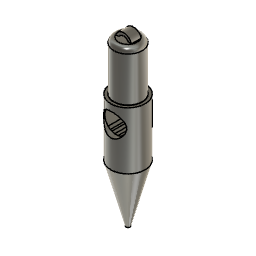
test nose cone v4 (Autodesk Fusion 360 design; units mm, degrees)
Autodesk Fusion 360 part; units mm, degrees
note: some values were not read from the file. Chosen so that the rebuilt part matches the saved one: which bodies a step acts on. Set by a fixed rule: which sketch regions a step uses.
sketch "Sketch1" plane through (0, 0, 0) normal (0, 1, 0) x (1, 0, 0)
  line L0 (-30, 466.4818) -> (-17.5, 473.5668)
  line L1 (0, 380) -> (0, 382.9635)
  line L2 (-14.4962, 382.9635) -> (0, 382.9635)
  line L3 (0, 550) -> (0, 382.9635)
  line L4 (-12.0481, 512.1856) -> (-35.0172, 529.9796)
  line L5 (-14.4962, 433) -> (-14.4962, 382.9635)
  line L6 (-18.356, 433) -> (-18.3, 433)
  line L7 (-17.5, 433.3365) -> (-14.5, 433.3365)
  arc A0 (-18.3, 433) -> (-18.5, 432.8) centre (-18.3, 432.8) ccw
  line L8 (-14.4962, 382.9635) -> (-14.4962, 433)
  line L9 (0, 382.9635) -> (0, 380)
  line L10 (17.5, 233) -> (-17.5, 233)
  line L11 (-14.4962, 397.7519) -> (-14.4962, 382.9635)
  line L12 (0, 382.9635) -> (0, 405)
  line L13 (-17.5, 433.3365) -> (-14.5, 433.3365)
  line L14 (-14.5, 433.3365) -> (-14.4962, 433)
  line L15 (0, 550) -> (-2, 550)
  line L16 (0, 550) -> (-2, 550)
  line L17 (-17.5, 456.7981) -> (-30, 466.4818)
  line L18 (0, 483.4858) -> (14.4363, 491.6682)
  line L19 (0, 382.9635) -> (-14.4962, 382.9635)
  line L20 (14.4363, 491.6682) -> (0, 502.8519)
  line L21 (-17.5, 433.3365) -> (-17.5, 491.6682)
  line L22 (-17.5, 491.6682) -> (-2, 550)
  line L23 (-14.4962, 382.9635) -> (-90, 460)
  line L24 (-90, 460) -> (-45.5915, 565.8682)
  line L25 (-45.5915, 565.8682) -> (-2, 550)
  constraint perpendicular L7 L21
  constraint coincident L21 L17.start
  constraint coincident L21 L0.end
  constraint coincident L22 L4.start
revolve "Revolve1" add sketch "Sketch1" angle 360 about axis through (0, 0, -382.9635) along (0, 0, 1) contours L2 L3 L5 L7 L8 L11 L12 L13 L14 L15 L16 L19 L21 L22 makes body 1
fillet "Fillet1" [no effect]
fillet "Fillet2" radius 5 1 edges at (-13.5152, 5.242, -382.9635) on bodies 1
ref_plane "WorkPlane1" through (0, 0, -382.9635) normal (0, 0, 1) x (1, 0, 0)
ref_plane "WorkPlane2" through (0, -14.4962, -421.9536) normal (0, -1, 0) x (1, 0, 0)
ref_plane "WorkPlane3" through (0, 0.5038, -421.9536) normal (0, -1, 0) x (1, 0, 0)
sketch "Sketch2" plane through (0, 0.5038, -421.9536) normal (0, -1, 0) x (1, 0, 0)
  arc A0 (5, 39) -> (-5, 39) centre (0, 36.3333) ccw
  arc A1 (8, 39) -> (-8, 39) centre (0, 36.6667) ccw
  line L0 (-8, 39) -> (-5, 39)
  line L1 (5, 39) -> (8, 39)
  constraint horizontal L0
  constraint parallel L0 L1
extrude "Extrude1" add sketch "Sketch2" along normal mid plane 10 separate body makes body 2
combine "Combine1" operation add target body 2 tool bodies 1 makes body 3 at (-17.4782, 0.8723, -452.7804)
combine "Combine2" operation add target body 2 tool bodies 3 makes body 4 at (-17.4782, 0.8723, -452.7804)
extrude "Extrude2" add 2 faces at (7, -1.1628, -382.9536) (-6, -1.1628, -382.9536) along direction (0, 0, -1) blind 5 on bodies 2 bodies 2 4
sketch "Sketch3" plane through (0, -14.4962, -421.9536) normal (0, -1, 0) x (1, 0, 0)
  line L0 (1.65, -43.7503) -> (7.65, -43.7503)
  line L1 (7.65, -41.5) -> (11.75, -41.5)
  line L2 (7.65, -43.7503) -> (7.65, -41.5)
  line L3 (1.65, -41.5) -> (1.65, -43.7503)
  line L4 (11.75, -41.5) -> (11.75, -18)
  line L5 (11.75, -18) -> (-11.75, -18)
  line L6 (-11.75, -18) -> (-11.75, -41.5)
  line L7 (-7.65, -41.5) -> (-7.65, -43.7503)
  line L8 (-15.75, -14) -> (15.75, -14)
  line L9 (-7.65, -43.7503) -> (-1.65, -43.7503)
  line L10 (15.75, -14) -> (15.75, -45.5)
  line L11 (-11.75, -41.5) -> (-7.65, -41.5)
  line L12 (-1.65, -43.7503) -> (-1.65, -41.5)
  line L13 (-15.75, -45.5) -> (-15.75, -14)
  line L14 (-1.65, -41.5) -> (1.65, -41.5)
  line L15 (15.75, -45.5) -> (-15.75, -45.5)
extrude "Extrude3" cut sketch "Sketch3" against normal blind 50 contours L0 L1 L2 L3 L4 L5 L6 L7 L9 L11 L12 L14 bodies 2
extrude "Extrude4" cut sketch "Sketch3" along normal blind 10 contours L0 L1 L2 L3 L4 L5 L6 L7 L9 L11 L12 L14 bodies 2
ref_plane "WorkPlane4" through (11.75, -12.9687, -439.9536) normal (0, -1, 0) x (1, 0, 0)
sketch "Sketch4" plane through (11.75, -12.9687, -439.9536) normal (0, -1, 0) x (1, 0, 0)
  line L0 (-23.5, -23.5) -> (-19.4, -23.5)
  line L1 (-23.5, -23.5) -> (-23.5, 0)
  line L2 (0, 0) -> (-23.5, 0)
  line L3 (0, 0) -> (0, -23.5)
  line L4 (-4.1, -23.5) -> (0, -23.5)
  line L5 (-4.1, -23.5) -> (-4.1, -25.7503)
  line L6 (-10.1, -25.7503) -> (-4.1, -25.7503)
  line L7 (-10.1, -25.7503) -> (-10.1, -23.5)
  line L8 (-13.4, -23.5) -> (-10.1, -23.5)
  line L9 (-13.4, -23.5) -> (-13.4, -25.7503)
  line L10 (-19.4, -25.7503) -> (-13.4, -25.7503)
  line L11 (-19.4, -25.7503) -> (-19.4, -23.5)
  line L12 (-10.1, -23.5) -> (-10.1, -25.7503)
  line L13 (-10.1, -25.7503) -> (-4.1, -25.7503)
  line L14 (-4.1, -25.7503) -> (-4.1, -23.5)
  line L15 (-4.1, -23.5) -> (0, -23.5)
  line L16 (0, -23.5) -> (0, 0)
  line L17 (0, 0) -> (-23.5, 0)
  line L18 (-23.5, 0) -> (-23.5, -23.5)
  line L19 (-23.5, -23.5) -> (-19.4, -23.5)
  line L20 (-19.4, -23.5) -> (-19.4, -25.7503)
  line L21 (-19.4, -25.7503) -> (-13.4, -25.7503)
  line L22 (-13.4, -25.7503) -> (-13.4, -23.5)
  line L23 (-13.4, -23.5) -> (-10.1, -23.5)
  line L24 (-29.25, 6.6171) -> (5.75, 6.6171)
  line L25 (-29.25, -51.7146) -> (5.75, -51.7146)
  line L26 (-23.5, 0) -> (0, 0)
  line L27 (0, 0) -> (0, -23.5)
  line L28 (0, -23.5) -> (-23.5, -23.5)
  line L29 (-23.5, -23.5) -> (-23.5, 0)
  line L30 (-23.5, 0) -> (-11.75, 0)
  line L31 (-11.75, 0) -> (-11.75, -23.5)
  circle A0 centre (-11.75, -11.75) radius 11.75
  constraint horizontal L26
  constraint vertical L27
  constraint horizontal L28
  constraint vertical L29
  constraint coincident L3.end L4.end
  constraint coincident L1.end L2.end
  constraint midpoint L26 L30.end
  constraint midpoint L8 L31.end
  constraint midpoint L31 A0.centre
  constraint coincident L30.end A0
extrude "Extrude5" add sketch "Sketch4" along normal blind 5 contours L0 L1 L8 L18 L19 L23 L28 L29 A0 | L9 L10 L11 L20 L21 L22 L28 | L1 L2 L17 L18 L26 L29 L30 A0 | L2 L3 L16 L17 L26 L27 A0 | L3 L4 L8 L15 L16 L23 L27 L28 A0 | L5 L6 L7 L12 L13 L14 L28 bodies 2
revolve "Revolve2" cut sketch "Sketch1" angle 360 about axis through (0, 0, -550) along (0, 0, 1) contours L0 L5 L7 L8 L11 L13 L14 L17 L21 L22 L23 L24 L25 | L0 L17 L21 bodies 2
extrude "Extrude6" add 4 faces at (10.8955, -12.9687, -459.7604) (-10.8955, -12.9687, -459.7604) (-9.4208, -12.9687, -442.2827) (9.4208, -12.9687, -442.2827) along direction (0, 1, 0) blind 1 on bodies 2 bodies 2
ref_plane "WorkPlane5" through (-5.875, 11.0313, -445.8286) normal (0, 1, 0) x (-1, 0, 0)
sketch "Sketch5" plane through (-5.875, 11.0313, -445.8286) normal (0, 1, 0) x (1, 0, 0)
  spline S0 degree 3 poles (5.875, -5.875) (5.1105, -5.875) (4.3276, -5.7992) (2.786, -5.4889) (2.0272, -5.2546) (-0.1352, -4.342) (-1.4233, -3.4437) (-3.4554, -1.4116) (-4.346, -0.1261) (-5.2531, 2.0237) (-5.4866, 2.7777) (-5.7976, 4.3166) (-5.875, 5.1016) (-5.875, 5.875) knots -1.845512 -1.845512 -1.845512 -1.845512 -1.616148 -1.616148 -1.386784 -1.386784 -0.928056 -0.928056 -0.464028 -0.464028 -0.232014 -0.232014 0 0 0 0
  spline S1 degree 3 poles (17.625, 5.875) (17.625, 5.1016) (17.5476, 4.3166) (17.2366, 2.7777) (17.0031, 2.0237) (16.096, -0.1261) (15.2054, -1.4116) (13.1733, -3.4437) (11.8852, -4.342) (9.7228, -5.2546) (8.964, -5.4889) (7.4224, -5.7992) (6.6395, -5.875) (5.875, -5.875) knots -3.691025 -3.691025 -3.691025 -3.691025 -3.459011 -3.459011 -3.226997 -3.226997 -2.762969 -2.762969 -2.304241 -2.304241 -2.074877 -2.074877 -1.845512 -1.845512 -1.845512 -1.845512
  spline S2 degree 3 poles (5.875, 17.625) (6.6395, 17.625) (7.4224, 17.5492) (8.964, 17.2389) (9.7228, 17.0046) (11.8852, 16.092) (13.1733, 15.1937) (15.2054, 13.1616) (16.096, 11.8761) (17.0031, 9.7263) (17.2366, 8.9723) (17.5476, 7.4334) (17.625, 6.6484) (17.625, 5.875) knots 1.845512 1.845512 1.845512 1.845512 2.074877 2.074877 2.304241 2.304241 2.762969 2.762969 3.226997 3.226997 3.459011 3.459011 3.691025 3.691025 3.691025 3.691025
  spline S3 degree 3 poles (-5.875, 5.875) (-5.875, 6.6484) (-5.7976, 7.4334) (-5.4866, 8.9723) (-5.2531, 9.7263) (-4.346, 11.8761) (-3.4554, 13.1616) (-1.4233, 15.1937) (-0.1352, 16.092) (2.0272, 17.0046) (2.786, 17.2389) (4.3276, 17.5492) (5.1105, 17.625) (5.875, 17.625) knots 0 0 0 0 0.232014 0.232014 0.464028 0.464028 0.928056 0.928056 1.386784 1.386784 1.616148 1.616148 1.845512 1.845512 1.845512 1.845512
  line L0 (7.525, 17.625) -> (7.525, 19.8753)
  line L1 (13.525, 19.8753) -> (7.525, 19.8753)
  line L2 (13.525, 19.8753) -> (13.525, 17.625)
  line L3 (17.625, 17.625) -> (13.525, 17.625)
  line L4 (17.625, 17.625) -> (17.625, -5.875)
  line L5 (-5.875, -5.875) -> (17.625, -5.875)
  line L6 (-5.875, -5.875) -> (-5.875, 17.625)
  line L7 (-1.775, 17.625) -> (-5.875, 17.625)
  line L8 (-1.775, 17.625) -> (-1.775, 19.8753)
  line L9 (4.225, 19.8753) -> (-1.775, 19.8753)
  line L10 (4.225, 19.8753) -> (4.225, 17.625)
  line L11 (7.525, 17.625) -> (4.225, 17.625)
  line L12 (23.375, -12.4921) -> (-11.625, -12.4921)
  line L13 (23.375, 45.8396) -> (-11.625, 45.8396)
extrude "Extrude7" add sketch "Sketch5" along normal blind 10 separate body makes body 5
sketch "Sketch6" plane through (0, 0, -433.3365) normal (0, 0, 1) x (-1, 0, 0)
  circle A0 centre (0, 0) radius 14.5
  circle A1 centre (0, 0) radius 17.5
  circle A2 centre (0, 0) radius 17.5
  line L0 (23.6136, -26.5135) -> (-23.6136, -26.5135)
  line L1 (-23.6136, -26.5135) -> (-23.6136, 26.5135)
  line L2 (-23.6136, 26.5135) -> (23.6136, 26.5135)
  line L3 (23.6136, 26.5135) -> (23.6136, -26.5135)
  line L4 (23.6136, -26.5135) -> (-23.6136, 26.5135) construction
  line L5 (-23.6136, -26.5135) -> (23.6136, 26.5135) construction
  constraint coincident A0.centre A1.centre
  constraint horizontal L0
  constraint perpendicular L0 L1
  constraint parallel L0 L2
  constraint parallel L1 L3
  constraint coincident L4 A0.centre
  constraint coincident L5 A0.centre
extrude "Extrude8" cut sketch "Sketch6" against normal blind 40 contours L0 L1 L2 L3 bodies 5
